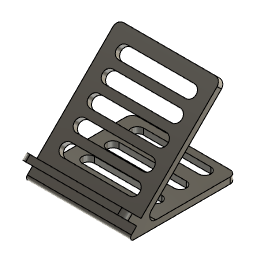
flip-5-stand v4 (Autodesk Fusion 360 design; units mm, degrees)
Autodesk Fusion 360 part; units mm, degrees
sketch "Sketch1" plane through (0, 0, 0) normal (1, 0, 0) x (0, 1, 0)
  line L0 (0, 0) -> (90, 0)
  line L1 (0, 0) -> (77.7817, 77.7817)
  line L2 (77.7817, 77.7817) -> (81.3173, 74.2462)
  line L3 (81.3173, 74.2462) -> (12.0711, 5)
  line L4 (12.0711, 5) -> (90, 5)
  line L5 (90, 5) -> (90, 0)
  dimension "d1" = 110
  dimension "d2" = 5
  dimension "d3" = 5
  dimension "d4" = 45
  dimension "d5" = 90
  constraint coincident L0.start L1.start
  constraint horizontal L0
  constraint perpendicular L1 L2
  constraint perpendicular L2 L3
  constraint horizontal L4
  constraint perpendicular L0 L5
  measures "d1" distance of L0.start L1.end
  measures "d2" distance of L0 L4
  measures "d3" distance of L1 L3
  measures "d4" angle of L3 L4
  measures "d5" distance of L0.start L0.end
extrude "Extrude1" add sketch "Sketch1" along normal blind 85
sketch "Sketch2" plane through (0, 0, 0) normal (0, -0.707107, 0.707107) x (1, 0, 0)
  line L0 (0, 110) -> (0, 0)
  line L1 (0, 0) -> (85, 0)
  line L2 (85, 0) -> (85, 110)
  line L3 (85, 110) -> (0, 110)
  line L4 (0, 12.0711) -> (85, 12.0711)
  line L5 (0, 0) -> (85, 0)
  line L6 (0, 17.0711) -> (85, 17.0711)
  line L7 (42.5, 17.0711) -> (42.5, 110) construction
  line L8 (42.5, 63.5355) -> (0, 63.5355) construction
  line L9 (15, 90) -> (70, 90)
  arc A0 (70, 90) -> (70, 100) centre (70, 95) ccw
  line L10 (70, 100) -> (15, 100)
  arc A1 (15, 100) -> (15, 90) centre (15, 95) ccw
  line L11 (15, 95) -> (70, 95) construction
  line L12 (70, 83.75) -> (15, 83.75)
  arc A2 (15, 83.75) -> (15, 73.75) centre (15, 78.75) ccw
  line L13 (15, 73.75) -> (70, 73.75)
  arc A3 (70, 73.75) -> (70, 83.75) centre (70, 78.75) ccw
  line L14 (70, 67.5) -> (15, 67.5)
  arc A4 (15, 67.5) -> (15, 57.5) centre (15, 62.5) ccw
  line L15 (15, 57.5) -> (70, 57.5)
  arc A5 (70, 57.5) -> (70, 67.5) centre (70, 62.5) ccw
  line L16 (70, 51.25) -> (15, 51.25)
  arc A6 (15, 51.25) -> (15, 41.25) centre (15, 46.25) ccw
  line L17 (15, 41.25) -> (70, 41.25)
  arc A7 (70, 41.25) -> (70, 51.25) centre (70, 46.25) ccw
  line L18 (70, 35) -> (15, 35)
  arc A8 (15, 35) -> (15, 25) centre (15, 30) ccw
  line L19 (15, 25) -> (70, 25)
  arc A9 (70, 25) -> (70, 35) centre (70, 30) ccw
  dimension "d8" = 5
  dimension "d51" = 10
  dimension "d52" = 10
  dimension "d53" = 10
  dimension "d54" = 5
  dimension "d57" = 0
  dimension "d58" = -65
  constraint coincident L0 L6.start
  constraint coincident L2 L6.end
  constraint perpendicular L2 L6
  constraint midpoint L6 L7.start
  constraint midpoint L3 L7.end
  constraint midpoint L7 L8.start
  constraint coincident L0 L8.end
  constraint perpendicular L0 L8
  constraint tangent L9 A0
  constraint tangent A0 L10
  constraint parallel L9 L10
  constraint tangent L10 A1
  constraint tangent L9 A1
  constraint parallel L3 L11
  measures "d8" distance of L4 L6
  measures "d51" distance of L3 L10
  measures "d52" distance of L0 A1
  measures "d53" distance of L2 A0
  measures "d54" radius of A0
extrude "Extrude2" add sketch "Sketch2" along normal blind 15 contours L0 L2 L4 L6
fillet "Fillet1" radius 2.5 1 edges at (42.5, 0, 0)
fillet "Fillet3" radius 5 1 edges at (42.5, 12.0711, 5)
fillet "Fillet4" radius 5 2 edges at (0, 79.5495, 76.014) (85, 79.5495, 76.014)
fillet "Fillet5" radius 5 2 edges at (85, -0.3033, 20.9099) (0, -0.3033, 20.9099)
sketch "Sketch3" plane through (0, 0, 5) normal (0, 0, 1) x (-1, 0, 0)
  line L0 (0, -24.1421) -> (-85, -24.1421)
  line L1 (-85, -24.1421) -> (-85, -90)
  line L2 (-85, -90) -> (0, -90)
  line L3 (0, -90) -> (0, -24.1421)
  line L4 (-42.5, -24.1421) -> (-42.5, -90) construction
  line L5 (-42.5, -57.0711) -> (-85, -57.0711) construction
  line L6 (-70, -44.1421) -> (-15, -44.1421)
  arc A0 (-15, -44.1421) -> (-15, -34.1421) centre (-15, -39.1421) ccw
  line L7 (-15, -34.1421) -> (-70, -34.1421)
  arc A1 (-70, -34.1421) -> (-70, -44.1421) centre (-70, -39.1421) ccw
  line L8 (-70, -39.1421) -> (-15, -39.1421) construction
  line L9 (-15, -54.1421) -> (-70, -54.1421)
  arc A2 (-70, -54.1421) -> (-70, -64.1421) centre (-70, -59.1421) ccw
  line L10 (-70, -64.1421) -> (-15, -64.1421)
  arc A3 (-15, -64.1421) -> (-15, -54.1421) centre (-15, -59.1421) ccw
  line L11 (-15, -74.1421) -> (-70, -74.1421)
  arc A4 (-70, -74.1421) -> (-70, -84.1421) centre (-70, -79.1421) ccw
  line L12 (-70, -84.1421) -> (-15, -84.1421)
  arc A5 (-15, -84.1421) -> (-15, -74.1421) centre (-15, -79.1421) ccw
  dimension "d61" = 10
  dimension "d62" = 10
  dimension "d63" = 10
  dimension "d64" = 5
  dimension "d67" = 0
  dimension "d68" = -40
  constraint midpoint L0 L4.start
  constraint midpoint L2 L4.end
  constraint midpoint L4 L5.start
  constraint midpoint L1 L5.end
  constraint tangent L6 A0
  constraint tangent A0 L7
  constraint parallel L6 L7
  constraint tangent L7 A1
  constraint tangent L6 A1
  constraint horizontal L8
  measures "d61" distance of L0 L7
  measures "d62" distance of L1 A1
  measures "d63" distance of L3 A0
  measures "d64" radius of A0
fillet "Fillet6" radius 5 2 edges at (85, 90, 2.5) (0, 90, 2.5)
sketch "Sketch4" plane through (0, 8.5355, 8.5355) normal (0, -0.707107, -0.707107) x (1, 0, 0)
  arc A0 (5, 15) -> (0, 10) centre (5, 10) ccw
  line L0 (0, 10) -> (0, 0)
  line L1 (85, 0) -> (85, 10)
  arc A1 (85, 10) -> (80, 15) centre (80, 10) ccw
  line L2 (80, 15) -> (5, 15)
  line L3 (9, 4.5) -> (76, 4.5)
  arc A2 (76, 4.5) -> (76, 12.5) centre (76, 8.5) ccw
  line L4 (76, 12.5) -> (9, 12.5)
  arc A3 (9, 12.5) -> (9, 4.5) centre (9, 8.5) ccw
  line L5 (9, 8.5) -> (76, 8.5) construction
  line L6 (0, 0) -> (85, 0)
  dimension "d43" = 5
  dimension "d44" = 5
  dimension "d47" = 8
  constraint tangent L3 A2
  constraint tangent A2 L4
  constraint parallel L3 L4
  constraint tangent L4 A3
  constraint tangent L3 A3
  constraint horizontal L5
  measures "d43" distance of L0 A3
  measures "d44" distance of L1 A2
  measures "d47" distance of L3 L4
extrude "Extrude5" cut sketch "Sketch4" against normal up to surface (5 mm away) contours L3 A2 L4 A3
extrude "Extrude6" cut sketch "Sketch2" against normal up to surface (5 mm away) contours L9 A0 L10 A1 | L12 A2 L13 A3 | L14 A4 L15 A5 | L16 A6 L17 A7 | L18 A8 L19 A9
extrude "Extrude7" cut sketch "Sketch3" against normal up to surface (5 mm away) contours L6 A0 L7 A1 | L9 A2 L10 A3 | L11 A4 L12 A5
named bodies: "flip-5-stand"
